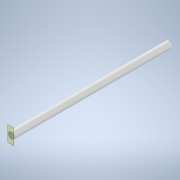
# Autodesk Inventor part: verticalRod
Saved by Autodesk Inventor 2022 (Build 260153000, 153)
## iProperties
Created: 2022-02-14
Part Number: verticalRod
Material: Generic
Document SubType Name: Modeling
Designer: tecware
Density: 1 g/cm^3
Appearance: Default
Author: tecware
Autodesk Inventor part; units mm, degrees
ref_plane "YZ Plane" through (0, 0, 0) normal (1, 0, 0) x (0, 1, 0)
ref_plane "XZ Plane" through (0, 0, 0) normal (0, 1, 0) x (-1, 0, 0)
ref_plane "XY Plane" through (0, 0, 0) normal (0, 0, 1) x (1, 0, 0)
ref_plane "Work Plane1" through (1.0442, 0, -99.0077) normal (0, 0, -1) x (-1, 0, 0)
sketch "Sketch1" plane through (1.0442, 0, -99.0077) normal (0, 0, -1) x (-1, 0, 0)
  circle A0 centre (1.0442, 0) radius 7.15
  point P0 (1.0442, 0)
  dimension "d0" = 14.3
  constraints: 1 centre point, 1 coincident
  measures "d0" diameter of A0
extrude "Extrusion1" add sketch "Sketch1" along normal blind 330
body "Solid1"
